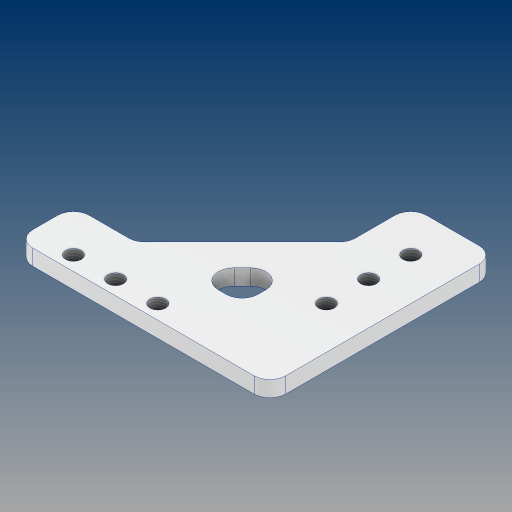
# Autodesk Inventor part: ELEV_006_SUPBRK1_THRD
Saved by Autodesk Inventor 2024.3 (Build 283343000, 343)
## iProperties
Created: 2024-11-25
Part Number: ELEV_006_SUPBRK1_THRD
Material: Aluminum 6061
Document SubType Name: Modeling
Designer: Kenji
Density: 2.7 g/cm^3
Appearance: Aluminum - Flat
Author: Kenji
Autodesk Inventor part; units mm, degrees
ref_plane "YZ Plane" through (0, 0, 0) normal (1, 0, 0) x (0, 1, 0)
ref_plane "XZ Plane" through (0, 0, 0) normal (0, 1, 0) x (-1, 0, 0)
ref_plane "XY Plane" through (0, 0, 0) normal (0, 0, 1) x (1, 0, 0)
sketch "Sketch1" plane through (0, 0, 0) normal (0, 1, 0) x (-1, 0, 0)
  line L0 (0, 7.112) -> (15.875, 7.112) construction
  line L1 (20.6375, -69.088) -> (4.7625, -69.088)
  line L2 (0, -64.3255) -> (0, -4.7625)
  line L3 (30.1625, -18.288) -> (76.2, -18.288) construction
  line L4 (76.2, -13.5255) -> (76.2, -4.7625)
  line L5 (71.4375, 0) -> (4.7625, 0)
  line L6 (25.4, -69.088) -> (25.4, -23.0505) construction
  arc A0 (30.1625, -18.288) -> (25.4, -23.0505) centre (30.1625, -23.0505) ccw construction
  arc A1 (0, -64.3255) -> (4.7625, -69.088) centre (4.7625, -64.3255) ccw
  arc A2 (76.2, -4.7625) -> (71.4375, 0) centre (71.4375, -4.7625) ccw
  arc A3 (4.7625, 0) -> (0, -4.7625) centre (4.7625, -4.7625) ccw
  circle A4 centre (12.7, -30.988) radius 2.3876
  circle A5 centre (12.7, -43.688) radius 2.3876
  circle A6 centre (12.7, -56.388) radius 2.3876
  circle A7 centre (63.5, -5.588) radius 2.3876
  circle A8 centre (50.8, -5.588) radius 2.3876
  circle A9 centre (38.1, -5.588) radius 2.3876
  line L7 (76.2, -5.588) -> (0, -5.588) construction
  line L8 (12.7, 0) -> (12.7, -69.088) construction
  line L9 (61.8117, -7.2763) -> (14.3883, -54.6997) construction
  line L10 (56.1403, -19.6829) -> (26.7949, -49.0283)
  line L11 (71.4375, -18.288) -> (59.5079, -18.288)
  line L12 (25.4, -52.3959) -> (25.4, -64.3255)
  arc A10 (71.4375, -18.288) -> (76.2, -13.5255) centre (71.4375, -13.5255) ccw
  arc A11 (20.6375, -69.088) -> (25.4, -64.3255) centre (20.6375, -64.3255) ccw
  arc A12 (59.5079, -18.288) -> (56.1403, -19.6829) centre (59.5079, -23.0505) ccw
  arc A13 (26.7949, -49.0283) -> (25.4, -52.3959) centre (30.1625, -52.3959) ccw
  line L13 (35.9347, -26.4181) -> (33.5301, -28.8227)
  line L14 (25.4, -25.4551) -> (25.4, -23.0505)
  line L15 (32.5671, -18.288) -> (30.1625, -18.288)
  arc A14 (30.1625, -18.288) -> (25.4, -23.0505) centre (30.1625, -23.0505) ccw
  arc A15 (35.9347, -26.4181) -> (32.5671, -18.288) centre (32.5671, -23.0505) ccw
  arc A16 (25.4, -25.4551) -> (33.5301, -28.8227) centre (30.1625, -25.4551) ccw
  point P0 (0, 0)
  point P1 (0, -69.088)
  point P2 (38.1, -5.588)
  point P3 (57.5352, -18.288)
  point P4 (25.4, -50.4232)
  point P5 (44.0648, -18.288)
  point P6 (25.4, -36.9528)
  dimension "d0" = 76.2
  dimension "d1" = 25.4
  dimension "d2" = 4.7625
  dimension "d3" = 4.7752
  dimension "d4" = 12.7
  dimension "d5" = 12.7
  dimension "d6" = 12.7
  dimension "d7" = 12.7
  dimension "d8" = 66.675
  dimension "d9" = 25.4
  dimension "d10" = 38.1
  dimension "d11" = 18.288
  dimension "d12" = 38.1
  dimension "d13" = 12.7
  dimension "d14" = 12.7
  dimension "d15" = 4.7625
  dimension "d16" = 4.7625
  dimension "d17" = 4.7625
  dimension "d18" = 4.7625
  constraints: 33 point on line, 32 end point, 22 point on circle, 22 tangent, 15 centre point, 10 equal radius, 5 parallel, 4 perpendicular, 3 horizontal, 3 midpoint, 2 collinear, 2 vertical, 1 coincident, 1 concentric, 8 other
  measures "d0" distance between parallel lines of L1 L0
  measures "d1" distance of point (25.4, -69.088) point (0, -69.088)
  measures "d2" radius of A0
  measures "d3" diameter of A4
  measures "d4" distance of point (12.7, -30.988) A5.centre
  measures "d5" distance of point (12.7, -56.388) A5.centre
  measures "d6" distance of A8.centre point (63.5, -5.588)
  measures "d7" distance of A9.centre A8.centre
  measures "d8" distance of L5.start L5.end
  measures "d9" distance from line of L0.start L3
  measures "d10" vertical distance of L0.start point (12.7, -30.988)
  measures "d11" distance between parallel lines of L3 L5
  measures "d12" distance from line of L2 A9.centre
  measures "d13" distance from line of L0.start L7
  measures "d14" distance between parallel lines of L2 L8
  measures "d15" distance between parallel lines of L9 L10
  measures "d16" radius of A10
  measures "d17" distance between parallel lines of L9 L13
  measures "d18" radius of A15
extrude "Extrusion1" add sketch "Sketch1" along normal blind 4.7625
thread "Thread1" size "10-32 UNF" class "2B" standard "ANSI Unified Screw Threads" full length
thread "Thread2" size "10-32 UNF" class "2B" standard "ANSI Unified Screw Threads" full length
thread "Thread3" size "10-32 UNF" class "2B" standard "ANSI Unified Screw Threads" full length
thread "Thread4" size "10-32 UNF" class "2B" standard "ANSI Unified Screw Threads" full length
thread "Thread5" size "10-32 UNF" class "2B" standard "ANSI Unified Screw Threads" full length
thread "Thread6" size "10-32 UNF" class "2B" standard "ANSI Unified Screw Threads" full length
sketch "Sketch2" plane through (0, 4.7625, 0) normal (0, 1, 0) x (1, 0, 0)
  line L0 (-71.4375, 0) -> (-4.7625, 0) projected
  line L1 (-76.2, 1.27) -> (0, 1.27)
  line L2 (-76.2, 13.5255) -> (-76.2, 4.7625) projected
  line L3 (0, 4.7625) -> (0, 64.3255) projected
  arc A0 (-4.7625, 0) -> (0, 4.7625) centre (-4.7625, 4.7625) ccw projected
  line L4 (-4.7625, 0) -> (0, 0)
  line L5 (0, 0) -> (0, 1.27)
  line L6 (-76.2, 1.27) -> (-76.2, 0)
  line L7 (-76.2, 0) -> (-71.4375, 0)
  point P0 (-1.5246, 1.27)
  dimension "d33" = 1.27
  constraints: 10 end point, 4 point on line, 2 perpendicular, 1 horizontal, 1 parallel, 1 tangent
  measures "d33" distance between parallel lines of L0 L1
extrude "Extrusion2" cut sketch "Sketch2" against normal through all contours L7 L6 L1 A0 L0
fillet "Fillet1" radius 4.7752 2 edges at (-74.6754, 2.3813, -1.27) (-1.5246, 2.3813, -1.27)
body "Solid1"
